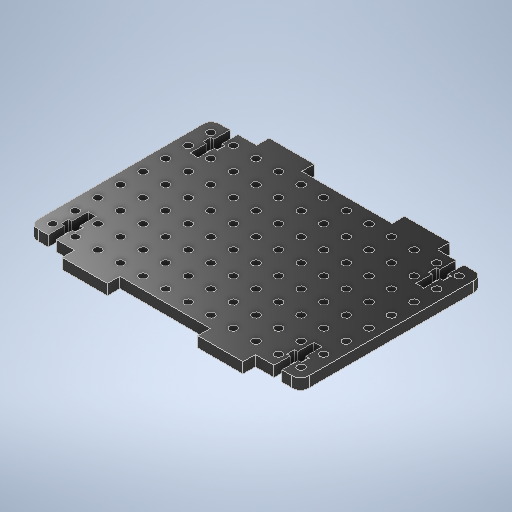
# Autodesk Inventor part: Mounting Base Side
Saved by Autodesk Inventor 2025.1 (Build 291241000, 241)
## iProperties
Created: 2024-05-30
Part Number: Mounting Base Side
Material: Polycarbonate, Smoke
Document SubType Name: Modeling
Designer: AlexForbes
Density: 1.2 g/cm^3
Appearance: Glossy - Black
Author: AlexForbes
Autodesk Inventor part; units mm, degrees
ref_plane "YZ Plane" through (0, 0, 0) normal (1, 0, 0) x (0, 1, 0)
ref_plane "XZ Plane" through (0, 0, 0) normal (0, 1, 0) x (-1, 0, 0)
sketch "Sketch1" plane through (0, 0, 0) normal (0, 1, 0) x (-1, 0, 0)
  line L0 (0, 0) -> (-152.4, 0)
  line L1 (-152.4, 0) -> (-152.4, -102.3)
  line L2 (-152.4, -102.3) -> (0, -102.3)
  line L3 (0, -102.3) -> (0, 0)
  dimension "d19" = 102.3
  dimension "d31" = 152.4
  constraints: 8 end point, 2 parallel, 1 horizontal, 1 perpendicular
  measures "d19" distance of L0.end L1.end
  measures "d31" distance of L1.end L2.end
extrude "Extrusion1" add sketch "Sketch1" along normal blind 6
ref_plane "Work Plane1" through (152.4, 0, -51.15) normal (0, 0, -1) x (-1, 0, 0)
sketch "Sketch3" plane through (0, 0, 0) normal (0, 1, 0) x (-1, 0, 0)
  line L0 (0, -102.3) -> (0, 0) projected
  line L1 (0, 0) -> (-152.4, 0) projected
  line L2 (-152.4, 0) -> (-152.4, -102.3) projected
  line L3 (-152.4, -102.3) -> (0, -102.3) projected
  line L4 (-25.4, -102.3) -> (-50.8, -102.3)
  line L5 (-50.8, -102.3) -> (-50.8, -109.3)
  line L6 (-50.8, -109.3) -> (-25.4, -109.3)
  line L7 (-25.4, -109.3) -> (-25.4, -102.3)
  line L8 (-101.6, -102.3) -> (-127, -102.3)
  line L9 (-127, -102.3) -> (-127, -109.3)
  line L10 (-127, -109.3) -> (-101.6, -109.3)
  line L11 (-101.6, -109.3) -> (-101.6, -102.3)
  line L12 (-101.6, -105.8) -> (-50.8, -105.8) construction
  line L13 (-152.4, -102.3) -> (0, -102.3) projected
  point P0 (-76.2, -102.3)
  point P1 (-50.8, -102.3)
  point P2 (-101.6, -102.3)
  point P3 (-127, -102.3)
  point P4 (-114.3, -109.3)
  point P5 (-38.1, -109.3)
  point P6 (-76.2, -105.8)
  point P7 (-76.2, -102.3)
  dimension "d20" = 7
  dimension "d32" = 76.2
  dimension "d33" = 25.4
  constraints: 18 end point, 7 midpoint, 4 parallel, 2 horizontal, 2 perpendicular, 2 point on line, 1 collinear, 1 horizontal alignment, 1 vertical alignment
  measures "d20" distance of L4.end L5.end
  measures "d32" distance of point (-114.3, -109.3) point (-38.1, -109.3)
  measures "d33" distance of L5.end L6.end
extrude "Extrusion2" add sketch "Sketch3" along normal up to surface (6 mm away) contours L7 L6 L5 L3 | L11 L10 L9 L3
mirror "Mirror1" about plane through (152.4, 0, -51.15) normal (0, 0, -1) of "Extrusion2"
sketch "Sketch4" plane through (0, 6, 0) normal (0, 1, 0) x (1, 0, 0)
  line L0 (73.9521, 22.5) -> (78.4479, 22.5) construction
  line L1 (72.075, 13.375) -> (72.075, 9.125) construction
  line L2 (80.325, 9.125) -> (80.325, 13.375) construction
  line L3 (73.9521, 0) -> (73.9521, 9.125) construction
  line L4 (73.9521, 13.375) -> (73.9521, 22.5) construction
  line L5 (78.4479, 22.5) -> (78.4479, 13.375) construction
  line L6 (78.4479, 9.125) -> (78.4479, 0) construction
  line L7 (80.325, 13.375) -> (78.4479, 13.375) construction
  line L8 (73.9521, 13.375) -> (72.075, 13.375) construction
  line L9 (72.075, 9.125) -> (73.9521, 9.125) construction
  line L10 (78.4479, 9.125) -> (80.325, 9.125) construction
  line L11 (73.9521, 0) -> (78.4479, 0) construction
  line L12 (50.8, 0) -> (101.6, 0) construction
  line L13 (10.4521, 22.5) -> (14.9479, 22.5)
  line L14 (10.4521, 13.375) -> (10.4521, 22.5)
  line L15 (8.575, 13.375) -> (8.575, 9.125)
  line L16 (10.4521, 0) -> (10.4521, 9.125)
  line L17 (16.825, 9.125) -> (16.825, 13.375)
  line L18 (8.575, 9.125) -> (10.4521, 9.125)
  line L19 (10.4521, 13.375) -> (8.575, 13.375)
  line L20 (14.9479, 9.125) -> (14.9479, 0)
  line L21 (14.9479, 22.5) -> (14.9479, 13.375)
  line L22 (16.825, 13.375) -> (14.9479, 13.375)
  line L23 (14.9479, 9.125) -> (16.825, 9.125)
  line L24 (10.4521, 0) -> (14.9479, 0)
  line L25 (137.4521, 22.5) -> (141.9479, 22.5)
  line L26 (137.4521, 13.375) -> (137.4521, 22.5)
  line L27 (135.575, 13.375) -> (135.575, 9.125)
  line L28 (137.4521, 0) -> (137.4521, 9.125)
  line L29 (143.825, 9.125) -> (143.825, 13.375)
  line L30 (135.575, 9.125) -> (137.4521, 9.125)
  line L31 (137.4521, 13.375) -> (135.575, 13.375)
  line L32 (141.9479, 9.125) -> (141.9479, 0)
  line L33 (141.9479, 22.5) -> (141.9479, 13.375)
  line L34 (143.825, 13.375) -> (141.9479, 13.375)
  line L35 (141.9479, 9.125) -> (143.825, 9.125)
  line L36 (137.4521, 0) -> (141.9479, 0)
  line L37 (0, 0) -> (25.4, 0) projected
  line L38 (127, 0) -> (152.4, 0) projected
  point P0 (76.2, 22.5)
  point P1 (76.2, 0)
  point P2 (12.7, 22.5)
  point P3 (139.7, 22.5)
  point P4 (12.7, 0)
  point P5 (139.7, 0)
  point P6 (139.7, 0)
  point P7 (12.7, 0)
  dimension "d24" = 22.5
  dimension "d25" = 4.25
  dimension "d26" = 8.25
  dimension "d28" = 4.4958
  dimension "d44" = 127
  constraints: 72 end point, 27 parallel, 20 equal length, 12 perpendicular, 11 midpoint, 6 horizontal alignment, 6 vertical, 3 horizontal, 3 vertical alignment
  measures "d24" distance of L0.end L6.end
  measures "d25" distance of L2.end L2.start
  measures "d26" distance of L2.start L1.end
  measures "d28" distance between parallel lines of L5 L4
  measures "d44" distance of point (139.7, 0) point (12.7, 0)
extrude "Extrusion3" cut sketch "Sketch4" against normal through all
fillet "Fillet1" radius 5 4 edges at (0, 3, 0) (152.4, 3, 0) (152.4, 3, -102.3) (0, 3, -102.3) curvature continuous yes
mirror "Mirror2" about plane through (152.4, 0, -51.15) normal (0, 0, -1) of "Extrusion3"
sketch "Sketch2" plane through (0, 6, 0) normal (0, 1, 0) x (1, 0, 0)
  line L0 (0, 0) -> (0, 6.7) construction
  line L1 (0, 6.7) -> (6.35, 6.7) construction
  line L2 (6.35, 6.7) -> (6.35, 0) construction
  line L3 (6.35, 0) -> (0, 0) construction
  dimension "d3" = 6.7
  dimension "d45" = 6.35
  constraints: 8 end point, 2 parallel, 1 coincident, 1 perpendicular, 1 vertical
  measures "d3" distance of L1.end L2.end
  measures "d45" distance of L0.end L1.end
hole "Hole1" at (6.35, 6, -6.7) direction (0, -1, 0) diameter 4.25 end through all
pattern_linear "Rectangular Pattern1" count 12 spacing 12.7 along (1, 0, 0) count 8 spacing 12.7 along (0, 0, -1) of "Hole1"
sketch "Sketch5" plane through (0, 6, 0) normal (0, 1, 0) x (1, 0, 0)
  circle A0 centre (31.75, 19.4) radius 2.125 construction
  circle A1 centre (31.75, 82.9) radius 2.125 construction
  line L0 (31.75, 19.4) -> (31.75, 82.9) construction
  circle A2 centre (6.35, 19.4) radius 2.125 construction
  point P0 (0, 0)
  dimension "d46" = 63.5
  dimension "d47" = 25.4
  constraints: 2 end point, 1 vertical
  measures "d46" distance of L0.start L0.end
  measures "d47" distance of A2.centre L0.start
body "Solid1"
